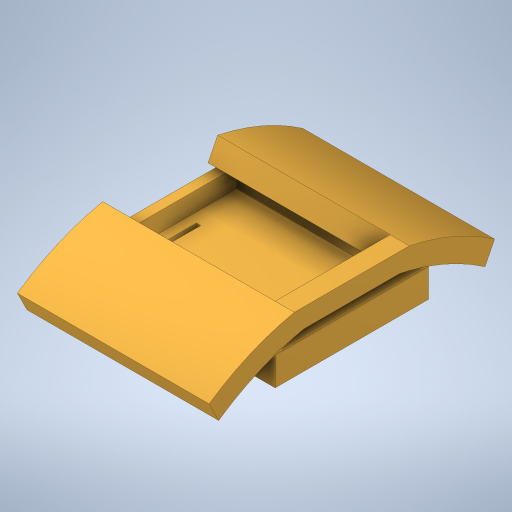
# Autodesk Inventor part: Part1
Saved by Autodesk Inventor 2024 (Build 280153000, 153)
## iProperties
Created: 2024-09-17
Part Number: Part1
Material: Generic
Document SubType Name: Modeling
Designer: domko
Density: 1 g/cm^3
Appearance: Brass - Satin
Author: domko
Autodesk Inventor part; units mm, degrees
ref_plane "YZ Plane" through (0, 0, 0) normal (1, 0, 0) x (0, 1, 0)
ref_plane "XZ Plane" through (0, 0, 0) normal (0, 1, 0) x (-1, 0, 0)
ref_plane "XY Plane" through (0, 0, 0) normal (0, 0, 1) x (1, 0, 0)
sketch "Sketch1" plane through (0, 0, 0) normal (0, 1, 0) x (-1, 0, 0)
  line L0 (50, 40) -> (-50, 40)
  line L1 (-50, 40) -> (-50, -40)
  line L2 (-50, -40) -> (50, -40)
  line L3 (50, -40) -> (50, 40)
  point P0 (0, 0)
  dimension "d0" = 40
  dimension "d1" = 80
  dimension "d2" = 100
  dimension "d3" = 50
  constraints: 8 end point, 2 parallel, 1 horizontal, 1 perpendicular
  measures "d0" distance from line of L2 point (0, 0)
  measures "d1" distance between parallel lines of L2 L0
  measures "d2" distance between parallel lines of L3 L1
  measures "d3" distance from line of L1 point (0, 0)
extrude "Extrusion1" add sketch "Sketch1" along normal blind 5
sketch "Sketch2" plane through (0, 5, 0) normal (0, 1, 0) x (1, 0, 0)
  line L0 (40, -8.89) -> (37.7775, -8.89)
  line L1 (37.7775, -8.89) -> (37.7775, 8.89)
  line L2 (37.7775, 8.89) -> (40, 8.89)
  line L3 (40, 8.89) -> (40, -8.89)
  line L4 (50, -40) -> (50, 40) projected
  point P0 (0, 0)
  point P1 (38.8888, -8.89)
  point P2 (38.8887, 8.89)
  point P3 (50, 0)
  point P4 (40, 0)
  dimension "d6" = 17.78
  dimension "d7" = 8.89
  dimension "d8" = 10
  dimension "d9" = 2.2225
  constraints: 8 end point, 4 midpoint, 2 parallel, 1 horizontal, 1 perpendicular
  measures "d6" distance of point (38.889, -8.89) point (38.889, 8.89)
  measures "d7" vertical distance of point (0, 0) point (38.889, 8.89)
  measures "d8" distance of point (50, 0) point (40, 0)
  measures "d9" distance between parallel lines of L3 L1
extrude "Extrusion2" cut sketch "Sketch2" against normal through all
sketch "Sketch3" plane through (0, 5, 0) normal (0, 1, 0) x (1, 0, 0)
  line L0 (-37.7775, -8.89) -> (-40, -8.89)
  line L1 (-40, -8.89) -> (-40, 8.89)
  line L2 (-40, 8.89) -> (-37.7775, 8.89)
  line L3 (-37.7775, 8.89) -> (-37.7775, -8.89)
  line L4 (-50, 40) -> (-50, -40) projected
  point P0 (0, 0)
  point P1 (-38.8887, -8.89)
  point P2 (-38.8887, 8.89)
  point P3 (-40, 0)
  dimension "d12" = 2.2225
  dimension "d13" = 8.89
  dimension "d14" = 17.78
  dimension "d15" = 10
  constraints: 8 end point, 3 midpoint, 2 parallel, 1 horizontal, 1 perpendicular
  measures "d12" distance between parallel lines of L1 L3
  measures "d13" distance from line of point (0, 0) L2
  measures "d14" distance of point (-38.889, -8.89) point (-38.889, 8.89)
  measures "d15" distance from line of L4 point (-40, 0)
extrude "Extrusion3" cut sketch "Sketch3" against normal through all
sketch "Sketch4" plane through (0, 5, 0) normal (0, 1, 0) x (1, 0, 0)
  line L0 (50, -40) -> (50, 40) projected
  line L1 (45, -35) -> (-45, -35)
  line L2 (-45, -35) -> (-45, 35)
  line L3 (-45, 35) -> (45, 35)
  line L4 (45, 35) -> (45, -35)
  line L5 (50, -40) -> (-50, -40)
  line L6 (-50, -40) -> (-50, 40)
  line L7 (-50, 40) -> (50, 40)
  line L8 (50, 40) -> (50, -40)
  dimension "d19" = 5
  dimension "d20" = 5
  dimension "d21" = 5
  dimension "d22" = 5
  constraints: 16 end point, 4 parallel, 2 horizontal, 2 perpendicular, 1 coincident
  measures "d19" distance between parallel lines of L4 L0
  measures "d20" distance between parallel lines of L5 L1
  measures "d21" distance between parallel lines of L6 L2
  measures "d22" distance between parallel lines of L7 L3
extrude "Extrusion4" add sketch "Sketch4" along normal blind 10
sketch "Sketch5" plane through (-50, 0, -40) normal (-1, 0, 0) x (0, 0, 1)
  line L0 (0, 0) -> (80, 0) projected
  line L1 (75, 15) -> (5, 15) projected
  arc A0 (109.4622, 0) -> (65, 19.1638) centre (40, -100) ccw
  arc A1 (15, 19.1638) -> (-29.4622, 0) centre (40, -100) ccw
  line L2 (15, 19.1638) -> (10, 29.1638)
  arc A2 (10, 29.1638) -> (-34.4622, 10) centre (35, -90) ccw
  line L3 (-29.4622, 0) -> (-34.4622, 10)
  arc A3 (114.4622, 10) -> (70, 29.1638) centre (45, -90) ccw
  line L4 (65, 19.1638) -> (70, 29.1638)
  line L5 (109.4622, 0) -> (114.4622, 10)
  point P0 (40, 0)
  point P1 (80, -100)
  point P2 (80, 15)
  point P3 (0, 15)
  point P4 (-5, 25)
  point P5 (85, 25)
  dimension "d25" = 100
  dimension "d26" = 100
  dimension "d27" = 15
  dimension "d28" = 15
  dimension "d29" = 15
  dimension "d30" = 10
  dimension "d31" = 5
  dimension "d32" = 5
  dimension "d33" = 15
  dimension "d34" = 10
  dimension "d35" = 10
  dimension "d36" = 10
  dimension "d37" = 10
  dimension "d38" = 5
  constraints: 12 point on circle, 8 end point, 4 centre point, 2 point on line, 1 coincident, 1 parallel
  measures "d25" distance from line of L0 point (80, -100)
  measures "d26" distance from line of L0 point (40, -100)
  measures "d27" horizontal distance of L2.start point (0, 15)
  measures "d28" horizontal distance of L4.start point (80, 15)
  measures "d29" horizontal distance of L2.end point (-5, 25)
  measures "d30" vertical distance of A2.centre A0.centre
  measures "d31" horizontal distance of L2.end L2.start
  measures "d32" horizontal distance of L3.start L3.end
  measures "d33" horizontal distance of L4.end point (85, 25)
  measures "d34" vertical distance of L2.end L2.start
  measures "d35" vertical distance of L3.end L3.start
  measures "d36" vertical distance of L5.end L5.start
  measures "d37" vertical distance of L4.end L4.start
  measures "d38" horizontal distance of L5.end L5.start
extrude "Extrusion5" add sketch "Sketch5" against normal blind 100
sketch "Sketch6" plane through (50, 0, 40) normal (1, 0, 0) x (0, 0, -1)
  arc A0 (114.4622, 10) -> (70, 29.1638) centre (45, -90) ccw projected
  line L0 (10, 29.1638) -> (70, 29.1638)
  arc A1 (80, 15) -> (65, 19.1638) centre (40, -100) ccw projected
  line L1 (15, 19.1638) -> (65, 19.1638)
  line L2 (65, 19.1638) -> (70, 29.1638)
  line L3 (15, 19.1638) -> (10, 29.1638)
  point P0 (40, 0)
  constraints: 8 end point, 2 coincident, 1 horizontal
extrude "Extrusion6" add sketch "Sketch6" against normal blind 10
body "Solid1"
